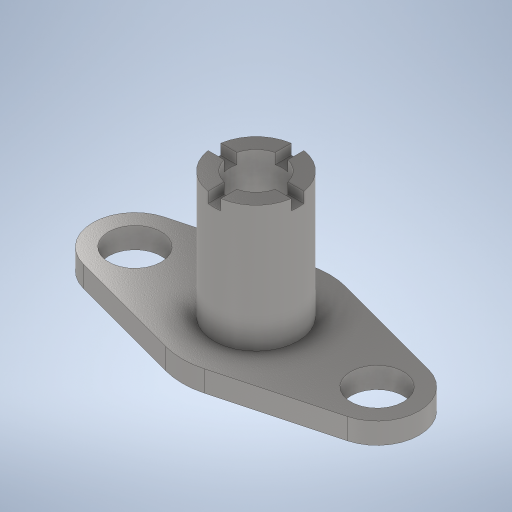
# Autodesk Inventor part: lager_
Saved by Autodesk Inventor 2024 (Build 280153000, 153)
## iProperties
Created: 2024-02-07
Part Number: lager_
Material: Stahl, galvanisiert
Document SubType Name: Modeling
Designer: ffogue
Density: 7.85 g/cm^3
Appearance: Galvanisiert
Author: ffogue
Autodesk Inventor part; units mm, degrees
ref_plane "YZ Plane" through (0, 0, 0) normal (1, 0, 0) x (0, 1, 0)
ref_plane "XZ Plane" through (0, 0, 0) normal (0, 1, 0) x (-1, 0, 0)
ref_plane "XY Plane" through (0, 0, 0) normal (0, 0, 1) x (1, 0, 0)
sketch "Skizze1" plane through (0, 0, 0) normal (0, 0, 1) x (1, 0, 0)
  circle A0 centre (0, 0) radius 20
  line L0 (-5.1764, 19.3185) -> (57.5, 36.1126)
  line L1 (-5.1764, -19.3185) -> (57.5, -36.1126)
  circle A1 centre (115, 0) radius 20
  line L2 (57.5, 36.1126) -> (120.1764, 19.3185)
  line L3 (57.5, -36.1126) -> (120.1764, -19.3185)
  circle A2 centre (115, 0) radius 12.5
  circle A3 centre (0, 0) radius 12.5
  dimension "d4" = 40
  dimension "d5" = 25
  dimension "d6" = 25
  dimension "d7" = 115
  dimension "d8" = 57.5
  dimension "d9" = 30
  dimension "d10" = 30
  constraints: 8 end point, 4 centre point, 4 point on circle, 3 coincident, 2 equal length, 2 tangent, 1 equal radius, 1 horizontal alignment, 1 vertical alignment
  measures "d4" diameter of A0
  measures "d5" diameter of A2
  measures "d6" diameter of A3
  measures "d7" distance of A1.centre A0.centre
  measures "d8" horizontal distance of L0.end A1.centre
  measures "d9" angle of L1 L0
  measures "d10" angle of L3 L2
extrude "Extrusion1" add sketch "Skizze1" along normal blind 10
sketch "Skizze2" plane through (0, 0, 10) normal (0, 0, 1) x (1, 0, 0)
  circle A0 centre (57.5, 0) radius 20
  point P0 (0, 0)
  point P1 (57.5, 36.1126)
  dimension "d13" = 40
  constraints: 1 centre point, 1 horizontal alignment, 1 vertical alignment
  measures "d13" diameter of A0
extrude "Extrusion2" add sketch "Skizze2" along normal blind 60
sketch "Skizze3" plane through (57.5, 0, 70) normal (0, 0, 1) x (1, 0, 0)
  circle A0 centre (0, 0) radius 20 projected
  line L0 (0, 0) -> (0, 5.5377) construction
  circle A1 centre (0, 0) radius 12.5
  point P0 (-57.5, 0)
  dimension "d17" = 25
  constraints: 2 end point, 1 centre point, 1 coincident, 1 vertical
  measures "d17" diameter of A1
extrude "Extrusion3" cut sketch "Skizze3" against normal up to surface (70 mm away) contours A1
sketch "Skizze4" plane through (57.5, 0, 70) normal (0, 0, 1) x (1, 0, 0)
  circle A0 centre (0, 0) radius 12.5 projected
  circle A1 centre (0, 0) radius 20 projected
  line L0 (-3, 19.7737) -> (-3, 12.1347)
  line L1 (3, 19.7737) -> (3, 12.1347)
  line L2 (0, 0) -> (0, 16.2882) construction
  circle A2 centre (0, 0) radius 20 projected
  point P0 (-57.5, 0)
  point P1 (3, 19.7737)
  dimension "d20" = 6
  constraints: 6 end point, 3 point on circle, 2 vertical, 1 parallel, 3 other
  measures "d20" distance between parallel lines of L1 L0
extrude "Extrusion4" cut sketch "Skizze4" against normal blind 5 contours A0 L0 A1 L1 picked at (-2.3362, 14.7892)
pattern_circular "Runde Anordnung1" count 4 over 360 about axis through (57.5, 0, 10) along (0, 0, 1) of "Extrusion4"
fillet "Rundung1" radius 35 2 edges at (57.5, 36.1126, 5) (57.5, -36.1126, 5)
equation "\"d6\" = d5"
